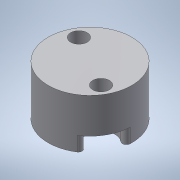
# Autodesk Inventor part: 06WX5378 / 25.105.3101.00
Saved by Autodesk Inventor 2020.3 (Build 243373000, 373)
## iProperties
RuleStatus: InUse
AfterDocSave0: file://Part Number Cleaner
Created: 2022-04-26
Material: Generic
Catalog Web Link: https://www.newark.com/pro-elec/25-105-3101-00/lamp-holder-dicr-gu5-3/dp/06WX5378
Vendor: NEWARK / MULTICOMP PRO
Document SubType Name: Modeling
Designer: solomone
Density: 1 g/cm^3
Appearance: Default
Part Number: 06WX5378 / 25.105.3101.00
LAB/DEPT: A. LEE (LAB)
DESIGN DEPARTMENT: HHMI: JRC - jET
ALTERED ITEM PART NUMBER: N/A
ALTERED ITEM VENDOR: N/A
ALTERED ITEM DESCRIPTION: N/A
Title: Standard
Author: solomone
Revision Number: 0
Autodesk Inventor part; units mm, degrees
ref_plane "YZ Plane" through (0, 0, 0) normal (1, 0, 0) x (0, 1, 0)
ref_plane "XZ Plane" through (0, 0, 0) normal (0, 1, 0) x (-1, 0, 0)
ref_plane "XY Plane" through (0, 0, 0) normal (0, 0, 1) x (1, 0, 0)
sketch "Sketch1" plane through (0, 0, 0) normal (0, 1, 0) x (-1, 0, 0)
  circle A0 centre (0, 0) radius 8.255
  dimension "d0" = 16.51
  constraints: 1 centre point, 1 coincident
  measures "d0" diameter of A0
extrude "Extrusion1" add sketch "Sketch1" along normal blind 9.8298
sketch "Sketch2" plane through (0, 0, 0) normal (0, -1, 0) x (1, 0, 0)
  line L0 (-5.1693, -2.9845) -> (5.1693, 2.9845) construction
  line L1 (-11.557, 0) -> (11.557, 0) projected
  point P0 (0, 0)
  dimension "d3" = 11.938
  dimension "d4" = 5.969
  dimension "d5" = 30
  constraints: 2 end point, 1 midpoint
  measures "d3" distance of L0.start L0.end
  measures "d4" distance of point (0, 0) L0.start
  measures "d5" angle of L1 L0
hole "Hole1" at (-5.1693, 0, -2.9845) at (5.1693, 0, 2.9845) direction (0, 1, 0) diameter 3.2766 end through all counterbore diameter 5.5626 counterbore depth 2.8448 clearance for "Socket Head Cap Screw" size "#4" standard "Ansi Unified Screw Threads"
fillet "Fillet1" radius 0.762 4 edges at (6.0414, 1.4224, 5.6255) (7.8926, 1.4224, 2.4192) (-6.0414, 1.4224, -5.6255) (-7.8926, 1.4224, -2.4192)
sketch "Sketch3" plane through (0, 0, 0) normal (0, -1, 0) x (1, 0, 0)
  point P0 (0, 0)
  point P1 (0, 2.5718)
  point P2 (0, -2.5718)
  dimension "d14" = 5.1435
  dimension "d15" = 2.5718
  constraints: 2 vertical alignment
  measures "d14" distance of point (0, -2.572) point (0, 2.572)
  measures "d15" distance of point (0, -2.572) point (0, 0)
hole "Hole2" at (0, 0, 2.5718) at (0, 0, -2.5718) direction (0, 1, 0) diameter 1.651 depth 5.08 tip angle 118
equation "\"d4\" = 0.5 * d3"
equation "\"d15\" = 0.5 * d14"
body "Solid1"
